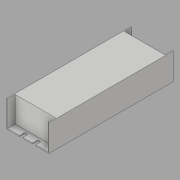
# Autodesk Inventor part: UHP-1500-230
Saved by Autodesk Inventor 2017 (Build 210142000, 142)
## iProperties
Created: 2022-09-19
Part Number: UHP-1500-230
Material: Generic
Document SubType Name: Modeling
Designer: JTS
Density: 1 g/cm^3
Appearance: Default
Author: JTS
Autodesk Inventor part; units mm, degrees
ref_plane "YZ Plane" through (0, 0, 0) normal (1, 0, 0) x (0, 1, 0)
ref_plane "XZ Plane" through (0, 0, 0) normal (0, 1, 0) x (-1, 0, 0)
sketch "Sketch1" plane through (0, 0, 0) normal (0, 0, 1) x (1, 0, 0)
  line L0 (-29.4, -18.5) -> (29.4, -18.5)
  line L1 (29.4, -18.5) -> (29.4, 18.5)
  line L2 (29.4, 18.5) -> (-29.4, 18.5)
  line L3 (-29.4, 18.5) -> (-29.4, -18.5)
  line L4 (-29.4, -18.5) -> (29.4, 18.5) construction
  line L5 (29.4, -18.5) -> (-29.4, 18.5) construction
  point P0 (0, 0)
  dimension "d0" = 58.8
  dimension "d1" = 37
  constraints: 12 end point, 2 horizontal, 2 midpoint, 2 vertical
  measures "d0" distance of L0.start L0.end
  measures "d1" distance of L2.end L0.start
extrude "Extrusion1" add sketch "Sketch1" along normal blind 173
sketch "Sketch2" plane through (-29.4, 18.5, 0) normal (0, 1, 0) x (1, 0, 0)
  line L0 (58.8, -173) -> (0, -173) projected
  line L1 (58.8, 0) -> (0, 0) projected
  arc A0 (22.65, -167.5) -> (18.15, -167.5) centre (20.4, -167.5) ccw
  arc A1 (40.65, -167.5) -> (36.15, -167.5) centre (38.4, -167.5) ccw
  arc A2 (36.15, -5.5) -> (40.65, -5.5) centre (38.4, -5.5) ccw
  arc A3 (18.15, -5.5) -> (22.65, -5.5) centre (20.4, -5.5) ccw
  line L2 (20.4, -167.5) -> (20.4, -5.5) construction
  line L3 (20.4, -5.5) -> (38.4, -5.5) construction
  line L4 (38.4, -5.5) -> (38.4, -167.5) construction
  line L5 (20.4, -167.5) -> (20.4, -173) construction
  line L6 (20.4, -5.5) -> (20.4, 0) construction
  line L7 (20.4, -5.5) -> (0, 0) construction
  line L8 (38.4, -5.5) -> (58.8, 0) construction
  line L9 (36.15, -167.5) -> (36.15, -173)
  line L10 (40.65, -167.5) -> (40.65, -173)
  line L11 (18.15, -167.5) -> (18.15, -173)
  line L12 (22.65, -167.5) -> (22.65, -173)
  line L13 (22.65, -5.5) -> (22.65, 0)
  line L14 (18.15, -5.5) -> (18.15, 0)
  line L15 (40.65, -5.5) -> (40.65, 0)
  line L16 (36.15, -5.5) -> (36.15, 0)
  point P0 (29.4, 0)
  dimension "d4" = 2.25
  dimension "d5" = 162
  dimension "d6" = 18
  constraints: 30 end point, 12 vertical, 10 point on line, 8 point on circle, 8 tangent, 4 centre point, 3 equal length, 3 equal radius, 1 coincident, 1 horizontal
  measures "d4" radius of A3
  measures "d5" distance of L2.start L2.end
  measures "d6" distance of L2.end L3.end
extrude "Extrusion2" cut sketch "Sketch2" against normal up to surface (37 mm away)
ref_plane "Work Plane1" through (29.4, -17.23, 0) normal (0, -1, 0) x (1, 0, 0)
sketch "Sketch3" plane through (-29.4, 18.5, 173) normal (0, 1, 0) x (1, 0, 0)
  line L0 (0, 173) -> (0, 0) projected
  line L1 (58.8, 173) -> (58.8, 0) projected
  line L2 (57.53, 0) -> (57.53, 10.5)
  line L3 (57.53, 10.5) -> (1.27, 10.5)
  line L4 (1.27, 10.5) -> (1.27, 0)
  line L5 (1.27, 0) -> (57.53, 0)
  line L6 (1.27, 0) -> (0, 0) construction
  line L7 (58.8, 0) -> (57.53, 0) construction
  line L8 (1.27, 162.5) -> (57.53, 162.5)
  line L9 (57.53, 162.5) -> (57.53, 173)
  line L10 (57.53, 173) -> (1.27, 173)
  line L11 (1.27, 173) -> (1.27, 162.5)
  line L12 (1.27, 173) -> (0, 173) construction
  point P0 (29.4, 173)
  dimension "d9" = 1.27
  dimension "d14" = 152
  constraints: 22 end point, 6 horizontal, 4 collinear, 2 vertical
  measures "d9" distance of L4.end L0.end
  measures "d14" distance between parallel lines of L8 L3
extrude "Extrusion3" cut sketch "Sketch3" against normal up to surface (35.73 mm away)
body "Solid1"
